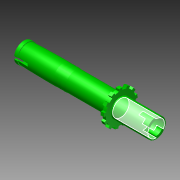
# Autodesk Inventor part: Motor Axle Connection
Saved by Autodesk Inventor 2015 (Build 190159000, 159)
## iProperties
Created: 2012-02-20
Part Number: Motor Axle Connection
Material: Generic
Document SubType Name: Modeling
Designer: Thom Tremblay
Density: 1 g/cm^3
Appearance: Dark Green
Author: Thom Tremblay
Autodesk Inventor part; units mm, degrees
ref_plane "YZ Plane" through (0, 0, 0) normal (1, 0, 0) x (0, 1, 0)
sketch "Sketch1" plane through (0, 0, 0) normal (0, 0, 1) x (1, 0, 0)
  line L0 (0, 0) -> (1.778, 0)
  line L1 (1.778, 0) -> (1.778, 5.08)
  line L2 (1.778, 5.08) -> (0, 5.08)
  line L3 (0, 5.08) -> (0, 0)
  line L4 (1.778, 0) -> (11.049, 0)
  line L5 (11.049, 0) -> (11.049, 3.683)
  line L6 (11.049, 3.683) -> (1.778, 3.683)
  line L7 (1.778, 3.683) -> (1.778, 0)
  line L8 (8.509, 3.683) -> (6.985, 3.81)
  line L9 (6.985, 3.81) -> (6.985, 3.683)
  line L10 (6.985, 3.683) -> (5.461, 3.81)
  line L11 (5.461, 3.81) -> (5.461, 3.683)
  line L12 (5.461, 3.683) -> (3.937, 3.81)
  line L13 (3.937, 3.81) -> (3.937, 3.683)
  line L14 (0, 0) -> (0, 3.125166)
  line L15 (0, 3.81) -> (0.889, 3.81) construction
  line L16 (0, 3.81) -> (0, 0)
  arc A0 (0, 3.81) -> (-9.906, 3.556) centre (0, -189.484) ccw
  line L17 (-9.906, 3.556) -> (-9.906, 3.81)
  line L18 (-9.906, 3.81) -> (-11.176, 3.81)
  line L19 (-11.176, 3.81) -> (-11.176, 0)
  line L20 (-11.176, 0) -> (0, 0)
  dimension "d0" = 1.778
  dimension "d1" = 10.16
  dimension "d2" = 9.271
  dimension "d3" = 7.366
  dimension "d4" = 7.62
  dimension "d5" = 2.54
  dimension "d6" = 1.524
  dimension "d7" = 7.62
  dimension "d8" = 7.62
  dimension "d9" = 11.176
  dimension "d10" = 7.112
  dimension "d11" = 1.27
  constraints: 42 end point, 8 parallel, 7 perpendicular, 6 point on line, 2 collinear, 2 horizontal, 2 horizontal alignment, 2 point on circle, 1 centre point, 1 tangent
  measures "d0" distance of L1.end L2.end
  measures "d1" diameter of L2 L0
  measures "d2" distance of L5.end L6.end
  measures "d3" diameter of L6 L4
  measures "d4" diameter of L8.end L4
  measures "d5" distance of L5.end L8.start
  measures "d6" horizontal distance of L8.start L8.end
  measures "d7" diameter of L18 L20
  measures "d8" diameter of L15 L20
  measures "d9" distance of L19.end L0.start
  measures "d10" diameter of L17.start L20
  measures "d11" distance of L17.end L18.end
sketch "Sketch1 outline for Revolution1" plane through (0, 0, 0) normal (0, 0, 1) x (1, 0, 0)
  line L0 (3.937, 3.81) -> (3.937, 3.683)
  line L1 (3.937, 3.683) -> (1.778, 3.683)
  line L2 (1.778, 3.683) -> (1.778, 5.08)
  line L3 (1.778, 5.08) -> (0, 5.08)
  line L4 (0, 5.08) -> (0, 3.81)
  arc A0 (0, 3.81) -> (-9.906, 3.556) centre (0, -189.484) ccw
  line L5 (-9.906, 3.556) -> (-9.906, 3.81)
  line L6 (-9.906, 3.81) -> (-11.176, 3.81)
  line L7 (-11.176, 3.81) -> (-11.176, 0)
  line L8 (-11.176, 0) -> (11.049, 0)
  line L9 (11.049, 0) -> (11.049, 3.683)
  line L10 (11.049, 3.683) -> (8.509, 3.683)
  line L11 (8.509, 3.683) -> (6.985, 3.81)
  line L12 (6.985, 3.81) -> (6.985, 3.683)
  line L13 (6.985, 3.683) -> (5.461, 3.81)
  line L14 (5.461, 3.81) -> (5.461, 3.683)
  line L15 (5.461, 3.683) -> (3.937, 3.81)
revolve "Revolution1" add sketch "Sketch1 outline for Revolution1" angle 360 about axis through (-11.176, 0, 0) along (1, 0, 0)
sketch "Sketch2" plane through (0, 0, 0) normal (0, 0, 1) x (1, 0, 0)
  line L0 (-11.176, 0.508) -> (-6.096, 0.508)
  line L1 (-6.096, 0.508) -> (-6.096, -0.508)
  line L2 (-6.096, -0.508) -> (-11.176, -0.508)
  line L3 (-11.176, -0.508) -> (-11.176, 0.508)
  line L4 (-11.176, -3.81) -> (-11.176, 3.81) construction
  point P0 (0, 0)
  point P1 (-11.176, 0)
  dimension "d13" = 1.016
  dimension "d14" = 5.08
  constraints: 8 end point, 2 midpoint, 2 parallel, 1 horizontal, 1 perpendicular
  measures "d13" distance of L2.end L0.start
  measures "d14" distance of L0.start L0.end
sketch "Sketch2 outline for Extrusion1" plane through (0, 0, 0) normal (0, 0, 1) x (1, 0, 0)
  line L0 (-11.176, 0.508) -> (-6.096, 0.508)
  line L1 (-6.096, 0.508) -> (-6.096, -0.508)
  line L2 (-6.096, -0.508) -> (-11.176, -0.508)
  line L3 (-11.176, -0.508) -> (-11.176, 0.508)
extrude "Extrusion1" cut sketch "Sketch2 outline for Extrusion1" along normal through all both and the other way through all
hole "Hole1" at (-11.176, 0, 0) direction (1, 0, 0) diameter 4.7625 depth 11.1125 counterbore diameter 6.35 counterbore depth 6.35
hole "Hole2" at (11.049, 0, 0) direction (-1, 0, 0) diameter 4.7625 depth 9.525 counterbore diameter 6.35 counterbore depth 1.27
sketch "Sketch3" plane through (1.778, 0, 0) normal (1, 0, 0) x (0, 0, -1)
  circle A0 centre (0, 0) radius 5.08 projected
  circle A1 centre (0, 0) radius 5.08
  circle A2 centre (0, 0) radius 3.683
  circle A3 centre (0, 0) radius 3.81 projected
  circle A4 centre (0, 0) radius 3.81
  circle A5 centre (0, 0) radius 3.81 projected
  circle A6 centre (0, 0) radius 3.683
  constraints: 4 centre point, 4 coincident, 2 concentric
sketch "Sketch3 outline for Extrusion2" plane through (1.778, 0, 0) normal (1, 0, 0) x (0, 0, -1)
  circle A0 centre (0, 0) radius 5.08
  circle A1 centre (0, 0) radius 3.81
extrude "Extrusion2" cut sketch "Sketch3 outline for Extrusion2" against normal blind 1.778
sketch "Sketch3 outline for Extrusion3" plane through (1.778, 0, 0) normal (1, 0, 0) x (0, 0, -1)
  circle A0 centre (0, 0) radius 3.81
  circle A1 centre (0, 0) radius 3.683
extrude "Extrusion3" add sketch "Sketch3 outline for Extrusion3" along normal blind 2.159
sketch "Sketch4" plane through (11.049, 0, 0) normal (1, 0, 0) x (0, 0, -1)
  circle A0 centre (0, 0) radius 3.683 projected
  circle A1 centre (0, 0) radius 3.175 projected
sketch "Sketch4 outline for Extrusion4" plane through (11.049, 0, 0) normal (1, 0, 0) x (0, 0, -1)
  circle A0 centre (0, 0) radius 3.683
  circle A1 centre (0, 0) radius 3.175
extrude "Extrusion4" add sketch "Sketch4 outline for Extrusion4" along normal blind 29.21
mirror "Mirror1" about plane through (40.259, 0, 0) normal (1, 0, 0) of "Revolution1", "Extrusion1", "Hole1", "Hole2", "Extrusion2", "Extrusion3", "Extrusion4"
ref_plane "Work Plane2" through (25.4, 0, 0) normal (-1, 0, 0) x (0, 0, 1)
sketch "Sketch7" plane through (25.4, 0, 0) normal (-1, 0, 0) x (0, 0, 1)
  circle A0 centre (0, 0) radius 5.715
  line L0 (0, 8.001) -> (0, -8.001)
  line L1 (0.635, 6.477) -> (-0.635, 6.477)
  line L2 (-0.635, 6.477) -> (-0.635, 5.679613)
  line L3 (-0.635, 5.461) -> (0, 5.461)
  line L4 (0.635, 5.679613) -> (0.635, 6.477)
  dimension "d43" = 11.43
  dimension "d44" = 0.635
  dimension "d45" = 0.635
  dimension "d46" = 0.254
  dimension "d47" = 0.762
  constraints: 8 end point, 2 parallel, 2 point on circle, 1 centre point, 1 coincident, 1 horizontal, 1 perpendicular, 1 point on line
  measures "d43" diameter of A0
  measures "d44" distance between parallel lines of L0 L2
  measures "d45" distance between parallel lines of L0 L4
  measures "d46" distance edge to line of A0 L3
  measures "d47" distance edge to line of A0 L1
sketch "Sketch7 outline for Extrusion5" plane through (25.4, 0, 0) normal (-1, 0, 0) x (0, 0, 1)
  arc A0 (-0.635, 5.679613) -> (0.635, 5.679613) centre (0, 0) ccw
  arc A1 (0.635, 5.679613) -> (-0.635, 5.679613) centre (0, 0) ccw
extrude "Extrusion5" add sketch "Sketch7 outline for Extrusion5" along normal mid plane 1.27
sketch "Sketch7 outline for Extrusion6" plane through (25.4, 0, 0) normal (-1, 0, 0) x (0, 0, 1)
  line L0 (0.635, 5.679613) -> (0.635, 6.477)
  arc A0 (-0.635, 5.679613) -> (0.635, 5.679613) centre (0, 0) cw
  line L1 (-0.635, 6.477) -> (-0.635, 5.679613)
  line L2 (0.635, 6.477) -> (-0.635, 6.477)
extrude "Extrusion6" add sketch "Sketch7 outline for Extrusion6" along normal mid plane 1.27
pattern_circular "Circular Pattern1" count 13 over 360 about axis through (25.4, 0, 0) along (-1, 0, 0) of "Extrusion6"
ref_plane "Work Plane3" through (34.544, 0, 0) normal (-1, 0, 0) x (0, 0, 1)
sketch "Sketch8" plane through (91.694, 0, 0) normal (1, 0, 0) x (0, 0, -1)
  circle A0 centre (0, 0) radius 10.040232
  constraints: 1 centre point, 1 coincident
sketch "Sketch8 outline for Extrusion7" plane through (91.694, 0, 0) normal (1, 0, 0) x (0, 0, -1)
  circle A0 centre (0, 0) radius 10.040232
extrude "Extrusion7" cut sketch "Sketch8 outline for Extrusion7" against normal up to surface (57.15 mm away)
sketch "Sketch9" plane through (0, 0, 0) normal (0, 0, 1) x (1, 0, 0)
  line L0 (26.035, 3.175) -> (34.544, 3.175)
  line L1 (26.035, 3.683) -> (34.544, 3.683)
  line L2 (26.035, -3.175) -> (34.544, -3.175)
  line L3 (26.035, -3.683) -> (34.544, -3.683)
  line L4 (34.430598, 2.667) -> (39.624, 2.667)
  line L5 (39.624, 2.667) -> (39.624, 3.175)
  line L6 (39.624, 3.175) -> (34.544, 3.175)
  line L7 (34.544, 3.175) -> (34.544, 3.683)
  line L8 (34.544, -3.175) -> (39.624, -3.175)
  line L9 (39.624, -3.175) -> (39.624, -3.683)
  line L10 (39.624, -3.683) -> (34.544, -3.683)
  line L11 (34.544, -3.683) -> (34.544, -3.175)
  line L12 (34.544, -3.175) -> (34.544, 3.175)
  line L13 (34.544, 0) -> (36.5125, 0) construction
  line L14 (34.544, 3.683) -> (39.624, 3.683)
  line L15 (39.624, 3.683) -> (39.624, 3.175)
  line L16 (39.624, 3.175) -> (34.544, 3.175)
  line L17 (34.544, 3.175) -> (34.544, 3.683)
  line L18 (39.624, -3.175) -> (34.544, -3.175)
  line L19 (34.544, -3.175) -> (34.544, -2.667)
  line L20 (34.544, -2.667) -> (39.624, -2.667)
  line L21 (39.624, -2.667) -> (39.624, -3.175)
  line L22 (34.544, 3.175) -> (34.544, 2.667)
  line L23 (39.624, 2.667) -> (39.624, 3.175)
  line L24 (34.544, 3.175) -> (34.544, 2.667)
  point P0 (0, 0)
  dimension "d58" = 5.08
  dimension "d59" = 5.08
  dimension "d62" = 0.508
  dimension "d63" = 0.508
  dimension "d64" = 5.08
  constraints: 40 end point, 7 parallel, 4 horizontal, 4 perpendicular, 3 point on line, 2 collinear, 1 midpoint
  measures "d58" distance of L5.end L6.end
  measures "d59" distance of L9.end L10.end
  measures "d62" distance of L4.end L5.end
  measures "d63" distance of L20.end L8.end
  measures "d64" distance of L7.end L14.end
sketch "Sketch9 outline for Revolution3" plane through (0, 0, 0) normal (0, 0, 1) x (1, 0, 0)
  line L0 (34.544, -3.175) -> (39.624, -3.175)
  line L1 (34.544, -2.667) -> (34.544, -3.175)
  line L2 (39.624, -2.667) -> (34.544, -2.667)
  line L3 (39.624, -3.175) -> (39.624, -2.667)
  line L4 (34.544, 3.175) -> (34.544, 2.667)
  line L5 (39.624, 3.175) -> (34.544, 3.175)
  line L6 (39.624, 2.667) -> (39.624, 3.175)
  line L7 (34.544, 2.667) -> (39.624, 2.667)
revolve "Revolution3" add sketch "Sketch9 outline for Revolution3" angle 60 about axis through (34.544, 0, 0) along (1, 0, 0)
sketch "Sketch9 outline for Revolution4" plane through (0, 0, 0) normal (0, 0, 1) x (1, 0, 0)
  line L0 (39.624, -3.175) -> (34.544, -3.175)
  line L1 (39.624, -3.683) -> (39.624, -3.175)
  line L2 (34.544, -3.683) -> (39.624, -3.683)
  line L3 (34.544, -3.175) -> (34.544, -3.683)
  line L4 (34.544, 3.683) -> (34.544, 3.175)
  line L5 (39.624, 3.683) -> (34.544, 3.683)
  line L6 (39.624, 3.175) -> (39.624, 3.683)
  line L7 (34.544, 3.175) -> (39.624, 3.175)
revolve "Revolution4" add sketch "Sketch9 outline for Revolution4" angle 360 about axis through (34.544, 0, 0) along (1, 0, 0)
sketch "Sketch10" plane through (0, 0, 0) normal (0, 1, 0) x (-1, 0, 0)
  line L0 (-26.035, -3.683) -> (-39.624, -3.683) projected
  line L1 (-26.035, 3.683) -> (-39.624, 3.683) projected
  line L2 (-26.035, 3.175) -> (-39.624, 3.175) projected
  line L3 (-39.624, 3.683) -> (-39.624, 0) projected
  line L4 (-49.784, 0) -> (21.336, 0) projected
  line L5 (-34.544, -3.175) -> (-37.084, -3.175)
  line L6 (-37.084, -3.175) -> (-37.084, -2.667)
  line L7 (-37.084, -2.667) -> (-34.544, -2.667)
  line L8 (-34.544, -2.667) -> (-34.544, -3.175)
  line L9 (-39.624, 0) -> (-39.624, -3.175) projected
  line L10 (-26.035, -3.175) -> (-39.624, -3.175) projected
  line L11 (-34.544, 3.175) -> (-37.084, 3.175)
  line L12 (-37.084, 3.175) -> (-37.084, 2.667)
  line L13 (-37.084, 2.667) -> (-34.544, 2.667)
  line L14 (-34.544, 2.667) -> (-34.544, 3.175)
  point P0 (0, 0)
  dimension "d69" = 0.508
  dimension "d70" = 2.54
  dimension "d71" = 5.08
  dimension "d72" = 0
  constraints: 16 end point, 4 symmetric about line, 2 parallel, 1 horizontal, 1 perpendicular
  measures "d69" distance of L7.end L5.start
  measures "d70" distance of L5.start L5.end
  measures "d71" distance between parallel lines of L9 L8
  measures "d72" distance between parallel lines of L10 L5
sketch "Sketch10 outline for Revolution5" plane through (0, 0, 0) normal (0, 1, 0) x (-1, 0, 0)
  line L0 (-34.544, -3.175) -> (-37.084, -3.175)
  line L1 (-37.084, -3.175) -> (-37.084, -2.667)
  line L2 (-37.084, -2.667) -> (-34.544, -2.667)
  line L3 (-34.544, -2.667) -> (-34.544, -3.175)
  line L4 (-37.084, 2.667) -> (-37.084, 3.175)
  line L5 (-37.084, 3.175) -> (-34.544, 3.175)
  line L6 (-34.544, 3.175) -> (-34.544, 2.667)
  line L7 (-34.544, 2.667) -> (-37.084, 2.667)
revolve "Revolution5" cut sketch "Sketch10 outline for Revolution5" angle 60 about axis through (0, 0, 0) along (-1, 0, 0)
sketch "Sketch14" plane through (37.084, 0, 0) normal (-1, 0, 0) x (0, 0.7071068, 0.7071068)
  circle A0 centre (0, 0) radius 3.683
  line L0 (-3.066814, 0.82175) -> (-2.576124, 0.69027)
  line L1 (-2.576124, 0.69027) -> (-3.066814, 0.82175)
  arc A1 (-2.576124, 0.69027) -> (-2.605627, 0.566696) centre (0.002483, 0.009335) ccw
  arc A2 (-3.066814, 0.82175) -> (-3.09723, 0.69842) centre (0, 0) ccw
  line L2 (-2.605627, 0.566696) -> (-3.09723, 0.69842)
  line L3 (-2.245064, -2.245064) -> (2.245064, 2.245064)
  line L4 (-0.666091, -0.666091) -> (-0.389236, -0.389236)
  line L5 (-2.605627, 0.566696) -> (-2.576124, 0.69027) construction
  dimension "d80" = 0.127
  constraints: 8 end point, 4 point on circle, 2 centre point, 2 point on line, 1 parallel
  measures "d80" distance between parallel lines of L0 L2
sketch "Sketch14 outline for Extrusion8" plane through (37.084, 0, 0) normal (-1, 0, 0) x (0, 0.7071068, 0.7071068)
  arc A0 (-2.605627, 0.566696) -> (-2.576124, 0.69027) centre (0.002483, 0.009335) cw
  line L0 (-3.09723, 0.69842) -> (-2.605627, 0.566696)
  arc A1 (-3.066814, 0.82175) -> (-3.09723, 0.69842) centre (0, 0) ccw
  line L1 (-2.576124, 0.69027) -> (-3.066814, 0.82175)
extrude "Extrusion8" add sketch "Sketch14 outline for Extrusion8" along normal blind 0.127
chamfer "Chamfer1" distance 0.127 angle 45 1 edges at (36.957, -1.4605, -2.5297)
sketch "Sketch15" plane through (37.084, 0, 0) normal (-1, 0, 0) x (0, 0.7071068, 0.7071068)
  line L0 (2.576124, -0.69027) -> (3.066814, -0.82175)
  arc A0 (2.576124, -0.69027) -> (1.885854, 1.885854) centre (0, 0) ccw
  circle A1 centre (0, 0) radius 3.175
  arc A2 (3.066814, -0.82175) -> (3.09723, -0.69842) centre (0, 0) ccw
  arc A3 (2.576124, -0.69027) -> (2.606072, -0.566815) centre (0, 0) ccw
  line L1 (3.066814, -0.82175) -> (2.576124, -0.69027)
  line L2 (2.606072, -0.566815) -> (3.09723, -0.69842)
  dimension "d79" = 0.127
  constraints: 6 point on circle, 4 end point, 3 concentric, 2 centre point, 1 collinear, 1 parallel
  measures "d79" distance between parallel lines of L2 L0
sketch "Sketch15 outline for Extrusion9" plane through (37.084, 0, 0) normal (-1, 0, 0) x (0, 0.7071068, 0.7071068)
  arc A0 (2.606072, -0.566815) -> (2.576124, -0.69027) centre (0, 0) cw
  line L0 (3.09723, -0.69842) -> (2.606072, -0.566815)
  arc A1 (3.066814, -0.82175) -> (3.09723, -0.69842) centre (0, 0) ccw
  line L1 (2.576124, -0.69027) -> (3.066814, -0.82175)
extrude "Extrusion9" add sketch "Sketch15 outline for Extrusion9" along normal blind 0.127
chamfer "Chamfer2" distance 0.127 angle 45 1 edges at (36.957, 1.4605, 2.5297)
equation "\"d8\" = d7"
body "Solid1"
